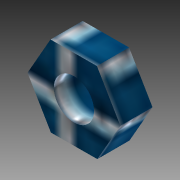
# Autodesk Inventor part: AA-Parafuso-M3-Porca
Saved by Autodesk Inventor 2014 SP1 (Build 180222100, 222)
## iProperties
Created: 2016-06-24
Part Number: AA-Parafuso-M3-Porca
Material: Genérico
Document SubType Name: Modeling
Designer: MarceloAdmin
Density: 1 g/cm^3
Appearance: Quadrado 1.5 pol - Azul médio
Author: MarceloAdmin
Autodesk Inventor part; units mm, degrees
ref_plane "YZ Plane" through (0, 0, 0) normal (1, 0, 0) x (0, 1, 0)
ref_plane "XZ Plane" through (0, 0, 0) normal (0, 1, 0) x (-1, 0, 0)
ref_plane "XY Plane" through (0, 0, 0) normal (0, 0, 1) x (1, 0, 0)
sketch "Esboço1" plane through (0, 0, 0) normal (0, 1, 0) x (-1, 0, 0)
  line L0 (1.716, -3.0092) -> (-1.7481, -2.9907)
  line L1 (-1.7481, -2.9907) -> (-3.4641, 0.0185)
  line L2 (-3.4641, 0.0185) -> (-1.716, 3.0092)
  line L3 (-1.716, 3.0092) -> (1.7481, 2.9907)
  line L4 (1.7481, 2.9907) -> (3.4641, -0.0185)
  line L5 (3.4641, -0.0185) -> (1.716, -3.0092)
  circle A0 centre (0, 0) radius 1.5
  dimension "d0" = 3
  dimension "d1" = 3
  constraints: 12 end point, 2 coincident, 1 centre point, 13 other
  measures "d0" diameter of A0
  measures "d1" distance from line of A0.centre L3
extrude "Extrusão1" add sketch "Esboço1" along normal blind 2.4
